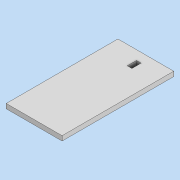
# Autodesk Inventor part: spiral base
Saved by Autodesk Inventor 2020 (Build 240168000, 168)
## iProperties
Created: 2020-12-17
Part Number: spiral base
Material: Generic
Document SubType Name: Modeling
Designer: solar
Density: 1 g/cm^3
Appearance: Default
Author: solar
Autodesk Inventor part; units mm, degrees
ref_plane "YZ Plane" through (0, 0, 0) normal (1, 0, 0) x (0, 1, 0)
ref_plane "XZ Plane" through (0, 0, 0) normal (0, 1, 0) x (-1, 0, 0)
ref_plane "XY Plane" through (0, 0, 0) normal (0, 0, 1) x (1, 0, 0)
sketch "Sketch1" plane through (0, 0, 0) normal (0, 1, 0) x (-1, 0, 0)
  circle A0 centre (0, 0) radius 10
  line L0 (0, -10) -> (0, -40)
  line L1 (0, -40) -> (0, -50)
  line L2 (0, -50) -> (-5, -50)
  line L3 (-5, -50) -> (-5, -40)
  line L4 (-5, -40) -> (0, -40)
  line L5 (-30, 0) -> (-30, -60)
  line L6 (-30, -60) -> (0, -60)
  line L7 (-30, -60) -> (30, -60)
  line L8 (30, -60) -> (30, 60)
  line L9 (30, 60) -> (-30, 60)
  line L10 (-30, 60) -> (-30, -60)
  dimension "d0" = 20
  dimension "d1" = 30
  dimension "d2" = 10
  dimension "d3" = 5
  dimension "d4" = 10
  dimension "d5" = 30
  dimension "d6" = 60
  dimension "d7" = 60
  dimension "d8" = 120
  constraints: 22 end point, 2 horizontal, 2 parallel, 2 perpendicular, 1 coincident, 1 point on line, 1 vertical, 1 vertical alignment, 2 other
  measures "d1" distance of L0.start L0.end
  measures "d2" distance of L0.end L1.end
  measures "d3" distance of L1.end L2.end
  measures "d4" distance of L2.end L3.end
  measures "d5" distance of L6.end L5.end
  measures "d6" distance of L5.end L5.start
  measures "d7" distance of L9.end L8.end
  measures "d8" distance of L8.end L7.end
extrude "Extrusion1" add sketch "Sketch1" along normal blind 5 contours A0 | L10 L9 L8 L7 L6 L5
body "Solid1"
